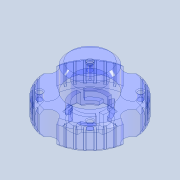
# Autodesk Inventor part: cpd_lowrcf_0.7_p2_v1
Saved by Autodesk Inventor 2021.2 (Build 252289000, 289)
## iProperties
Created: 2021-12-07
Part Number: cpd_lowrcf_0.7_p2_v1
Material: Generic
Document SubType Name: Modeling
Designer: tomos
Density: 1 g/cm^3
Appearance: Clear - Blue
Author: tomos
Autodesk Inventor part; units mm, degrees
ref_plane "YZ Plane" through (0, 0, 0) normal (1, 0, 0) x (0, 1, 0)
ref_plane "XZ Plane" through (0, 0, 0) normal (0, 1, 0) x (-1, 0, 0)
ref_plane "XY Plane" through (0, 0, 0) normal (0, 0, 1) x (1, 0, 0)
sketch "Sketch1" plane through (0, 0, 0) normal (0, 0, 1) x (1, 0, 0)
  line L0 (0, 0) -> (0, 7.0545) construction
  line L1 (0, 0) -> (4.1333, 0) construction
  line L2 (0.385, 0) -> (0.385, 3.65)
  line L3 (12.5, -10) -> (4.05, -10)
  line L4 (4.05, -10) -> (4.05, 0)
  line L5 (4.05, 0) -> (0.385, 0)
  line L6 (6.425, 4.65) -> (6.425, -3.05)
  line L7 (6.425, -3.05) -> (12.5, -3.05)
  line L8 (12.5, -3.05) -> (12.5, -10)
  line L9 (0.385, 3.65) -> (0.6495, 3.65)
  line L10 (0.6495, 3.65) -> (0.6845, 4.65)
  line L11 (0.6845, 4.65) -> (6.425, 4.65)
  dimension "d0" = 0.385
  dimension "d2" = 4.05
  dimension "d8" = 10
  dimension "d9" = 6.425
  dimension "d10" = 12.5
  dimension "d59" = 0.6495
  dimension "d60" = 2
  dimension "d65" = 1
  dimension "d66" = 4.65
  dimension "d67" = 7.7
  constraints: 24 end point, 4 perpendicular, 3 horizontal, 2 point on line, 2 vertical, 1 collinear
  measures "d0" distance between parallel lines of L2 L0
  measures "d2" distance between parallel lines of L4 L0
  measures "d8" distance between parallel lines of L3 L1
  measures "d9" distance between parallel lines of L6 L0
  measures "d10" distance between parallel lines of L8 L0
  measures "d59" distance from line of L0 L9.end
  measures "d60" angle of L0 L10
  measures "d65" distance between parallel lines of L9 L11
  measures "d66" distance between parallel lines of L1 L11
  measures "d67" distance between parallel lines of L7 L11
revolve "Revolution1" add sketch "Sketch1" angle 360 about axis through (0, 0, 0) along (0, 1, 0)
chamfer "Chamfer2" distance 1 angle 45 3 edges at (-6.425, 4.65, 0) (-12.5, -3.05, 0) (-12.5, -10, 0)
sketch "Sketch3" plane through (0, -10, 0) normal (0, -1, 0) x (1, 0, 0)
  circle A0 centre (0, 0) radius 4
  circle A1 centre (0, 0) radius 5.2
  circle A2 centre (0, 0) radius 11.5 construction
  line L0 (0, 0) -> (0, -10.6084) construction
  line L1 (-1.2, -3.8158) -> (-1.2, -5.0596)
  line L2 (1.2, -3.8158) -> (1.2, -5.0596)
  point P0 (1.2, -3.8158)
  dimension "d17" = 8
  dimension "d18" = 10.4
  dimension "d19" = 1.2
  constraints: 6 end point, 3 coincident, 2 symmetric about line, 2 vertical, 6 other
  measures "d19" distance between parallel lines of L1 L0
extrude "Extrusion1" cut sketch "Sketch3" against normal blind 4.2 contours A0 L2 A1 L1 picked at (-0.9352, -4.2849)
sketch "Sketch4" plane through (0, 0, 0) normal (1, 0, 0) x (0, 1, 0)
  line L0 (0, 0) -> (-13.7637, 0) construction
  line L1 (0, 0) -> (0, -5.6642) construction
  line L2 (0, -4) -> (-17.2907, -4) construction
  line L3 (-8.1, -4) -> (-5.8, -4)
  line L4 (-5.8, -4) -> (-5.8, -5.2)
  line L5 (-5.8, -5.2) -> (-8.1, -5.2)
  line L6 (-8.1, -5.2) -> (-8.1, -4)
  dimension "d22" = 4
  dimension "d23" = 5.8
  dimension "d24" = 1.2
  dimension "d25" = 2.3
  constraints: 14 end point, 3 horizontal, 2 parallel, 2 point on line, 1 perpendicular, 1 vertical
  measures "d22" distance between parallel lines of L2 L0
  measures "d23" distance between parallel lines of L1 L4
  measures "d24" distance between parallel lines of L5 L2
  measures "d25" distance between parallel lines of L4 L6
revolve "Revolution2" cut sketch "Sketch4" angle 60 about axis through (0, 0, 0) along (0, 1, 0)
pattern_circular "Circular Pattern1" count 4 over 360 about axis through (0, -10, 0) along (0, 1, 0) of "Extrusion1", "Revolution2"
chamfer "Chamfer3" distance 1 angle 45 16 edges at (2.8638, -10, 2.8638) (4.4639, -10, 1.2) (5.2, -10, 0) (4.4639, -10, -1.2) (2.8638, -10, -2.8638) (1.2, -10, -4.4639) (0, -10, -5.2) (-1.2, -10, -4.4639) (-2.8638, -10, -2.8638) (-4.4639, -10, -1.2) (-5.2, -10, 0) (-4.4639, -10, 1.2) (-2.8638, -10, 2.8638) (-1.2, -10, 4.4639) (0, -10, 5.2) (1.2, -10, 4.4639)
sketch "Sketch5" plane through (0, -10, 0) normal (0, -1, 0) x (1, 0, 0)
  circle A0 centre (0, 0) radius 12.5
  circle A1 centre (0, 0) radius 12
  line L0 (0, 0) -> (-3.6414, 0) construction
  line L1 (-11.9974, 0.25) -> (-12.4975, 0.25)
  line L2 (-11.9974, -0.25) -> (-12.4975, -0.25)
  point P0 (-12.4975, -0.25)
  point P1 (-12.2474, -0.25)
  dimension "d34" = 25
  dimension "d35" = 24
  dimension "d33" = 0.25
  constraints: 6 end point, 4 coincident, 2 horizontal, 2 symmetric about line, 6 other
  measures "d33" distance between parallel lines of L1 L0
extrude "Extrusion2" cut sketch "Sketch5" against normal through all contours L1 A1 L2 A0 picked at (-12.1649, 0.1944)
pattern_circular "Circular Pattern2" count 36 over 360 about axis through (0, -10, 0) along (0, 1, 0) of "Extrusion2"
sketch "Sketch6" plane through (0, -3.05, 0) normal (0, 1, 0) x (1, 0, 0)
  circle A0 centre (0, 0) radius 12.5
  circle A1 centre (0, 0) radius 0.385 construction
  line L0 (0, 0) -> (0, 16.4064) construction
  circle A2 centre (0, 12.5) radius 2.5
  point P0 (-2.4875, 12.25)
  point P1 (2.4875, 12.25)
  dimension "d41" = 25
  dimension "d42" = 5
  constraints: 2 end point, 1 centre point, 1 coincident, 1 point on line, 1 vertical, 3 other
  measures "d42" diameter of A2
extrude "Extrusion3" cut sketch "Sketch6" against normal through all contours A2 A0 picked at (0, 11.6481)
pattern_circular "Circular Pattern3" count 4 over 360 about axis through (0, -10, 0) along (0, 1, 0) of "Extrusion3"
sketch "Sketch7" plane through (0, -3.05, -12.5) normal (0, 1, 0) x (1, 0, 0)
  circle A0 centre (0, -12.5) radius 0.385 construction
  circle A1 centre (0, -12.5) radius 10.5 construction
  line L0 (0, -12.5) -> (-15.963, -12.5) construction
  line L1 (0, -12.5) -> (-12.3969, -0.1031) construction
  circle A2 centre (-7.4246, -5.0754) radius 0.8
  dimension "d48" = 21
  dimension "d49" = 45
  dimension "d50" = 1.6
  constraints: 4 end point, 1 centre point, 1 coincident, 1 horizontal, 1 point on line, 3 other
  measures "d49" angle of L1 L0
  measures "d50" diameter of A2
extrude "Extrusion4" cut sketch "Sketch7" against normal blind 2
chamfer "Chamfer4" distance 0.25 angle 45 1 edges at (-8.2246, -3.05, -7.4246)
pattern_circular "Circular Pattern4" count 4 over 360 about axis through (0, -10, 0) along (0, 1, 0) of "Extrusion4", "Chamfer4"
chamfer "Chamfer5" distance 0.25 angle 45 1 edges at (-0.6845, 4.65, 0)
equation "\"d8\" = pedestal_height"
equation "\"d66\" = rotor_length"
equation "\"pedestal_height\" = 10"
equation "\"rotor_diameter\" = 0.7"
equation "\"tolerancefactor\" = 1.1"
equation "\"rotor_length\" = 4.65"
equation "\"cutpipette_enddiameter\" = 1.181"
body "Solid1"
